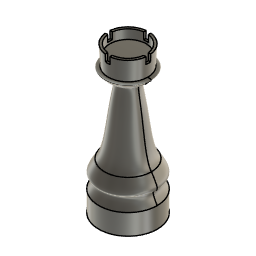
rook (Autodesk Fusion 360 design; units mm, degrees)
Autodesk Fusion 360 part; units mm, degrees
sketch "Sketch1" plane through (0, 0, 0) normal (0, 1, 0) x (1, 0, 0)
  line L0 (4.127, 0) -> (12.7, 0)
  line L1 (0, -8.1) -> (0, -63.5)
  line L2 (4.127, -8.1) -> (4.127, 0)
  line L3 (4.127, -8.1) -> (0, -8.1)
  line L4 (12.7, 0) -> (12.7, -8.89)
  spline S0 degree 5 poles (12.7, -8.89) (12.5228, -9.1703) (12.1908, -9.7112) (11.7599, -10.4632) (11.3204, -11.347) (10.996, -12.2534) (10.8908, -12.9659) (10.9891, -13.4977) (11.2597, -13.8749) (11.6519, -14.1397) (12.0871, -14.3585) (12.4688, -14.6121) (12.7087, -14.9729) (12.7446, -15.489) (12.5687, -16.1589) (12.2271, -16.9325) (11.7934, -17.7351) (11.3515, -18.4845) (10.9729, -19.1112) (10.6997, -19.5749) (10.5166, -19.8911) (10.3941, -20.0731) (10.2872, -20.1975) (10.2046, -20.2793) (10.1606, -20.32) knots 0 0 0 0 0 0 0.05 0.1 0.15 0.2 0.25 0.3 0.35 0.4 0.45 0.5 0.55 0.6 0.65 0.7 0.75 0.8 0.85 0.9 0.95 1 1 1 1 1 1
  line L5 (11.0164, -19.5298) -> (9.3048, -21.1102)
  line L6 (10.1606, -20.32) -> (10.1606, -20.3182)
  spline S1 degree 5 poles (10.1606, -20.3182) (10.072, -20.4282) (9.8974, -20.6638) (9.6429, -21.0647) (9.3185, -21.694) (8.938, -22.6383) (8.5822, -23.7377) (8.2506, -24.986) (7.942, -26.3718) (7.6548, -27.8771) (7.3864, -29.4786) (7.134, -31.1494) (6.8942, -32.8611) (6.6636, -34.5859) (6.4383, -36.2982) (6.2147, -37.9767) (5.9891, -39.6061) (5.7578, -41.1797) (5.5189, -42.6968) (5.274, -44.158) (5.0305, -45.5618) (4.8039, -46.9) (4.6194, -48.1537) (4.514, -49.2901) (4.5409, -50.2548) (4.756, -50.9869) (5.1871, -51.4515) (5.8151, -51.6624) (6.5339, -51.7224) (7.1898, -51.7947) (7.6806, -52.0304) (8.0264, -52.504) (8.469, -53.1586) (9.1297, -53.8697) (10.0265, -54.495) (10.3039, -54.933) (9.6389, -55.1218) (9.0841, -55.1814) (8.7596, -55.1874) (8.6096, -55.182) knots 0 0 0 0 0 0 0.028571 0.057143 0.085714 0.114286 0.142857 0.171429 0.2 0.228571 0.257143 0.285714 0.314286 0.342857 0.371429 0.4 0.428571 0.457143 0.485714 0.514286 0.542857 0.571429 0.6 0.628571 0.657143 0.685714 0.714286 0.742857 0.771429 0.8 0.828571 0.857143 0.885714 0.914286 0.942857 0.971429 1 1 1 1 1 1
  line L7 (7.5916, -52.046) -> (12.232, -56.9275)
  line L8 (13.974, -55.3761) -> (3.2452, -54.9878)
  line L9 (8.6096, -55.182) -> (8.9358, -63.5)
  line L10 (8.9358, -63.5) -> (0, -63.5)
  point P0 (11.43, -13.97)
  point P1 (12.7, -15.24)
  point P2 (10.8683, -19.2903)
  point P3 (9.9118, -54.4867)
  point P4 (7.5916, -52.046)
  point P5 (5.4659, -51.5103)
  point P6 (6.1525, -38.4157)
  point P7 (8.1897, -25.2994)
  point P8 (4.59, -48.5898)
  dimension "d1" = 12.7
  dimension "d2" = 63.5
  dimension "d5" = 8.89
  dimension "d9" = 4.127
  dimension "d10" = 8.1
  constraint horizontal L0
  constraint perpendicular L0 L1
  constraint perpendicular L0 L2
  constraint perpendicular L1 L3
  constraint perpendicular L0 L4
  constraint midpoint S0.end L5
  constraint vertical L6
  constraint midpoint P3 L7
  constraint midpoint S1.end L8
  constraint coincident P4 L7.start
  measures "d1" distance of origin L0.end
  measures "d2" distance of origin L1.end
  measures "d5" distance of L0.end L4.end
  measures "d9" distance of L1.start L2.start
  measures "d10" distance of L0.start L2.start
revolve "Revolve1" add sketch "Sketch1" angle 360 about axis through (0, 0, 8.1) along (0, 0, 1) contours L0 L1 L2 L3 L4 S0 S1 L7 L9 L10 | S1 L7 picked at (7.8071, -52.2644)
sketch "CrownIndent" plane through (0, 0, 63.5) normal (0, 0, 1) x (-1, 0, 0)
  line L0 (-1, -8.9358) -> (-1, -8.8797) construction
  line L1 (-1, -7.8365) -> (-1, -10.89)
  line L2 (1, -7.8365) -> (1, -10.89)
  line L3 (-8.9358, 0) -> (0, 0)
  line L4 (1, 7.8365) -> (1, 10.89)
  line L5 (-1, 7.8365) -> (-1, 10.89)
  line L6 (7.8365, -1) -> (10.89, -1)
  line L7 (7.8365, 1) -> (10.89, 1)
  line L8 (-7.8365, -1) -> (-10.89, -1)
  line L9 (-7.8365, 1) -> (-10.89, 1)
  arc A0 (-1, -10.89) -> (1, -10.89) centre (0, 0) ccw
  arc A1 (-10.89, 1) -> (-10.89, -1) centre (0, 0) ccw
  arc A2 (10.89, -1) -> (10.89, 1) centre (0, 0) ccw
  arc A3 (1, 10.89) -> (-1, 10.89) centre (0, 0) ccw
  circle A4 centre (0, 0) radius 7.9
  dimension "d15" = 15.8
  constraint parallel L0 L1
  constraint coincident L1.end A2
  constraint symmetric L2.end L3 L4.end
  constraint symmetric L1.end L3 L5.end
  constraint concentric A0 A2
  constraint concentric A1 A2
  constraint concentric A2 A3
  constraint coincident A4 L7.start
  constraint coincident A4 L6.start
  constraint coincident A4 L5.start
  constraint coincident A4 L4.start
  constraint coincident A4 L8.start
  constraint coincident A4 L9.start
  constraint coincident A4 L2.start
  constraint coincident A4 L1.start
  constraint coincident L1 L0.end
  measures "d15" diameter of A4
extrude "Extrude1" cut sketch "CrownIndent" against normal blind 3 contours A4
extrude "Extrude2" cut sketch "CrownIndent" against normal blind 3 contours L1 L2 A0 A4 | L8 L9 A1 A4 | L6 L7 A2 A4 | L4 L5 A3 A4
extrude "Extrude3" cut sketch "CrownIndent" against normal blind 4 contours A4
